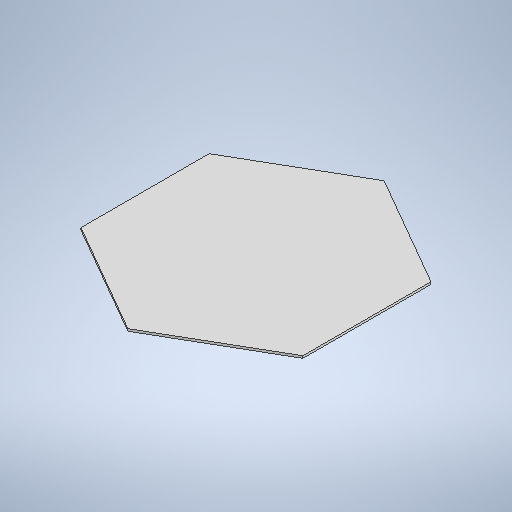
# Autodesk Inventor part: DSB 126 hex cup
Saved by Autodesk Inventor 2025 (Build 290162010, 162A)
## iProperties
Created: 2024-12-09
Part Number: DSB 126 hex cup
Material: Stainless Steel
Document SubType Name: Sheet Metal
Designer: user
Mass: 543.227 g
Surface Area: 692.751 cm^2
Volume: 67.9033 cm^3
Density: 8 g/cm^3
Sheet Metal Rule: AISI304 4mm Die 32
Sheet Metal Width: 198,000 mm
Sheet Metal Length: 228,631 mm
Sheet Metal Area: 45268,880 mm^2
Appearance: Default
Flat Pattern Width: 19.8 cm
Flat Pattern Length: 22.8631 cm
Flat Pattern Area: 452.689 cm^2
Octaeder_side: 55.919 mm
Octaeder_flange_lenth: 72.500 mm
Author: user
Autodesk Inventor part; units mm, degrees
ref_plane "YZ Plane" through (0, 0, 0) normal (1, 0, 0) x (0, 1, 0)
ref_plane "XZ Plane" through (0, 0, 0) normal (0, 1, 0) x (-1, 0, 0)
ref_plane "XY Plane" through (0, 0, 0) normal (0, 0, 1) x (1, 0, 0)
sketch "Sketch8" plane through (0, 0, 0) normal (0, 0, 1) x (1, 0, 0)
  circle A0 centre (0, 0) radius 82
  line L0 (99, -57.1577) -> (0, -114.3154)
  line L1 (0, -114.3154) -> (-99, -57.1577)
  line L2 (-99, -57.1577) -> (-99, 57.1577)
  line L3 (-99, 57.1577) -> (0, 114.3154)
  line L4 (0, 114.3154) -> (99, 57.1577)
  line L5 (99, 57.1577) -> (99, -57.1577)
  dimension "d44" = 164
  dimension "d47" = 198
  measures "d44" diameter of A0
  measures "d47" distance between parallel lines of L5 L2
extrude "Plate3" add sketch "Sketch8" along normal blind 2 contours A0 | L0 L1 L2 L3 L4 L5
equation "\"d48\" = Thickness"
equation "\"BendReliefWidth\" = Thickness"
equation "\"BendReliefDepth\" = 0.5 * Thickness"
equation "\"CornerReliefSize\" = 4 * Thickness"
equation "\"MinimumRemnant\" = 2 * Thickness"
equation "\"TransitionRadius\" = BendRadius"
equation "\"JacobiRadiusSize\" = BendRadius"
equation "\"GapSize\" = Thickness"
equation "\"Octaeder_side\" = d41"
equation "\"Octaeder_flange_lenth\" = d42"
equation "\"Thickness\" = 2"
equation "\"BendRadius\" = 6"
equation "\"d41\" = 55.918831"
equation "\"d42\" = 72.5"
body "Solid2"
